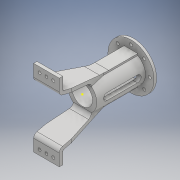
# Autodesk Inventor part: Standard
Saved by Autodesk Inventor 2017 (Build 210142000, 142)
## iProperties
Created: 2018-11-18
Part Number: Standard
Material: Generic
Document SubType Name: Modeling
Designer: Arman Grewal
Density: 1 g/cm^3
Appearance: Default
Author: Arman Grewal
Autodesk Inventor part; units mm, degrees
ref_plane "YZ Plane" through (0, 0, 0) normal (1, 0, 0) x (0, 1, 0)
ref_plane "XZ Plane" through (0, 0, 0) normal (0, 1, 0) x (-1, 0, 0)
sketch "Sketch1" plane through (0, 0, 0) normal (1, 0, 0) x (0, 1, 0)
  line L0 (-60, -12) -> (-60, 12)
  line L1 (-60, -13.0507) -> (-60, -12)
  arc A0 (-37.1036, -17) -> (-48.7347, -18.3716) centre (-37.1036, -67) ccw
  line L2 (-60, -12) -> (-3, -12)
  line L3 (-1, -12) -> (-60, -12)
  line L4 (-3, -17) -> (-37.1036, -17)
  line L5 (-3, 27) -> (-3, -27)
  line L6 (-3, -12) -> (-3, -17)
  line L7 (-102, -45) -> (-102, -30.9493)
  line L8 (-98.1581, -26.0853) -> (-63.8419, -17.9147)
  arc A1 (-63.8419, -17.9147) -> (-60, -13.0507) centre (-65, -13.0507) ccw
  line L9 (-96.4652, -29.788) -> (-48.7347, -18.3716)
  arc A2 (-96.4652, -29.788) -> (-98, -31.7331) centre (-96, -31.7331) ccw
  line L10 (-98, -45) -> (-98, -31.7331)
  arc A3 (-98.1581, -26.0853) -> (-102, -30.9493) centre (-97, -30.9493) ccw
  line L11 (-102, -45) -> (-98, -45)
  point P0 (0, 0)
  point P1 (0, 0)
  point P2 (0, 0)
  point P3 (-43, -17)
  point P4 (-60, -16)
  point P5 (-3, -16)
  point P6 (-102, -27)
  dimension "d0" = 18
  dimension "d1" = 40
  dimension "d2" = 4
  dimension "d3" = 2
  dimension "d4" = 5
  dimension "d5" = 50
  dimension "d6" = 13.451
  dimension "d7" = 166.608
  dimension "d8" = 33
  dimension "d9" = 5
  dimension "d10" = 38
  dimension "d11" = 57
  dimension "d12" = 12
  dimension "d13" = 3
  dimension "d14" = 12
  dimension "d15" = 3
  dimension "d16" = 12
  dimension "d17" = 3
  dimension "d18" = 2
  dimension "d19" = 39
  dimension "d20" = 4
  dimension "d21" = 0
  dimension "d22" = 15
  dimension "d23" = 24
  dimension "d24" = 57
  dimension "d25" = 4
  dimension "d26" = 57
  constraints: 24 end point, 8 point on circle, 8 tangent, 7 point on line, 4 centre point, 2 perpendicular, 2 vertical, 1 equal radius, 1 horizontal, 1 parallel
  measures "d0" distance of L7.start point (-102, -27)
  measures "d1" distance of L4.start point (-43, -17)
  measures "d2" distance of L7.start L10.start
  measures "d3" radius of A2
  measures "d4" radius of A3
  measures "d5" radius of A0
  measures "d6" angle of L3 L9
  measures "d7" angle of L3 L8
  measures "d8" distance between parallel lines of L3 L11
  measures "d9" distance between parallel lines of L3 L4
  measures "d10" distance between parallel lines of L0 L10
  measures "d11" distance between parallel lines of L6 L1
  measures "d12" distance from line of point (0, 0) L3
  measures "d13" distance from line of point (0, 0) L6
  measures "d14" distance from line of point (0, 0) L3
  measures "d15" distance from line of point (0, 0) L6
  measures "d16" distance from line of point (0, 0) L3
  measures "d17" distance from line of point (0, 0) L6
  measures "d18" distance from line of L3.start L6
  measures "d19" distance from line of L5.start L3
  measures "d20" distance from line of point (-3, -16) L3
  measures "d21" distance from line of point (-3, -16) L6
  measures "d22" distance from line of L5.end L3
  measures "d23" distance from line of L0.end L3
  measures "d24" distance from line of L3.end L6
  measures "d25" distance from line of point (-60, -16) L3
  measures "d26" distance from line of point (-60, -16) L6
extrude "Extrusion1" add sketch "Sketch1" along normal mid plane 30
mirror "Mirror1" about plane through (0, 0, 0) normal (0, 0, 1) of "Extrusion1"
sketch "Sketch2" plane through (-15, -3, -12) normal (0, 1, 0) x (1, 0, 0)
  circle A0 centre (15, -12) radius 27
  circle A1 centre (15, -12) radius 12
  dimension "d29" = 54
  dimension "d30" = 24
  dimension "d31" = 0
  constraints: 2 centre point, 2 coincident
  measures "d29" diameter of A0
  measures "d30" diameter of A1
  measures "d31" distance of point (15, -12) A0.centre
extrude "Extrusion2" add sketch "Sketch2" along normal blind 3
sketch "Sketch3" plane through (0, 0, 0) normal (0, 1, 0) x (1, 0, 0)
  circle A0 centre (-22, 0) radius 1.75
  circle A1 centre (-15.5563, -15.5563) radius 1.75
  circle A2 centre (0, -22) radius 1.75
  circle A3 centre (15.5563, -15.5563) radius 1.75
  circle A4 centre (22, 0) radius 1.75
  circle A5 centre (15.5563, 15.5563) radius 1.75
  circle A6 centre (0, 22) radius 1.75
  circle A7 centre (-15.5563, 15.5563) radius 1.75
  arc A8 (-21.9304, -1.7486) -> (-16.7436, -14.2707) centre (0, 0) ccw
  arc A9 (-16.7436, 14.2707) -> (-21.9304, 1.7486) centre (0, 0) ccw
  arc A10 (-1.7486, 21.9304) -> (-14.2707, 16.7436) centre (0, 0) ccw
  arc A11 (14.2707, 16.7436) -> (1.7486, 21.9304) centre (0, 0) ccw
  arc A12 (21.9304, 1.7486) -> (16.7436, 14.2707) centre (0, 0) ccw
  arc A13 (1.7486, -21.9304) -> (14.2707, -16.7436) centre (0, 0) ccw
  dimension "d36" = 3.5
  dimension "d37" = 360
  dimension "d39" = 22
  dimension "d40" = 22
  dimension "d41" = 22
  dimension "d42" = 22
  dimension "d43" = 22
  dimension "d44" = 22
  dimension "d45" = 22
  dimension "d46" = 22
  dimension "d48" = 6.4436
  dimension "d49" = 22
  constraints: 20 point on circle, 10 centre point, 1 coincident, 29 other
  measures "d36" diameter of A0
  measures "d39" radius of A13
  measures "d40" radius of A12
  measures "d41" radius of A11
  measures "d42" radius of A10
  measures "d43" radius of A9
  measures "d44" radius of A8
  measures "d45" distance of point (0, 0) point (22, 0)
  measures "d46" distance of point (0, 0) A12.start
  measures "d48" vertical distance of A5.centre A6.centre
  measures "d49" distance of point (0, 0) A5.centre
extrude "Extrusion3" cut sketch "Sketch3" against normal blind 3
sketch "Sketch4" plane through (0, 0, 0) normal (0, 1, 0) x (1, 0, 0)
  circle A0 centre (0, 0) radius 14
  circle A1 centre (0, 0) radius 12
  dimension "d52" = 28
  dimension "d53" = 24
  dimension "d54" = 0
  constraints: 2 centre point, 2 coincident
  measures "d52" diameter of A0
  measures "d53" diameter of A1
  measures "d54" distance of point (0, 0) A0.centre
extrude "Extrusion4" cut sketch "Sketch4" against normal blind 1
ref_plane "Work Plane1" through (0, 0, -45.25) normal (0, 0, 1) x (1, 0, 0)
sketch "Sketch6" plane through (0, 0, -45.25) normal (0, 0, 1) x (1, 0, 0)
  line L0 (-15, -102) -> (15, -102)
  line L1 (15, -102) -> (15, -88)
  line L2 (15, -96.4652) -> (15, -48.7347)
  line L3 (-15, -98.1581) -> (-15, -102)
  line L4 (-15, -102) -> (-15, -88)
  line L5 (-15, -48.7347) -> (-15, -96.4652)
  line L6 (15, -102) -> (-15, -102)
  line L7 (15, -88) -> (15, -43)
  line L8 (15, -43) -> (-15, -43)
  line L9 (-15, -43) -> (-15, -88)
  line L10 (0, -43) -> (-8, -43)
  line L11 (-8, -43) -> (8, -43)
  line L12 (15, -88) -> (8, -43)
  line L13 (-8, -43) -> (-15, -88)
  line L14 (8, -43) -> (8, -3)
  line L15 (-27, -3) -> (27, -3)
  line L16 (-8, -3) -> (-8, -43)
  line L17 (15, -43) -> (15, -3)
  line L18 (8, -3) -> (-15, -3)
  line L19 (-15, -43) -> (-15, -3)
  line L20 (-8, -43) -> (-8, -3)
  line L21 (-15, -3) -> (-15, -43)
  line L22 (-16.5227, -48) -> (-16.5227, -12)
  line L23 (-8, -43) -> (-15, -43)
  line L24 (-15, -37.1036) -> (-15, -48.7347)
  point P0 (0, 0)
  point P1 (0, 0)
  dimension "d71" = 14
  dimension "d72" = 45
  dimension "d73" = 8
  dimension "d74" = 16
  dimension "d75" = 8.842
  dimension "d76" = 8.842
  dimension "d77" = 8.842
  dimension "d78" = 90
  dimension "d79" = 8.842
  dimension "d80" = 8.842
  dimension "d81" = 8.842
  dimension "d82" = 31.5227
  dimension "d83" = 40
  dimension "d84" = 15
  dimension "d85" = 1.2955
  dimension "d86" = 12
  dimension "d87" = 6.0354
  dimension "d88" = 1.3012
  dimension "d89" = 15
  dimension "d90" = 1.2955
  dimension "d91" = 21.8204
  dimension "d92" = 23.6081
  dimension "d93" = 30.9447
  dimension "d94" = 31.2049
  dimension "d95" = 19.4664
  dimension "d96" = 24.9998
  dimension "d97" = 42
  constraints: 50 end point, 9 point on line, 5 parallel, 3 perpendicular, 2 collinear, 1 horizontal, 1 midpoint, 1 vertical
  measures "d71" distance of L0.end L1.end
  measures "d72" distance of L1.end L17.start
  measures "d73" distance of L10.start L16.end
  measures "d74" distance of L16.end L14.start
  measures "d75" angle of L17 L12
  measures "d76" angle of L17 L13
  measures "d77" angle of L7 L12
  measures "d78" angle of L18 L1
  measures "d79" angle of L5 L12
  measures "d80" angle of L4 L12
  measures "d81" angle of L3 L12
  measures "d82" distance between parallel lines of L17 L22
  measures "d83" distance between parallel lines of L15 L8
  measures "d84" distance from line of point (0, 0) L17
  measures "d85" distance from line of point (0, 0) L12
  measures "d86" distance from line of L15.end L17
  measures "d87" distance from line of L2.end L12
  measures "d88" distance from line of L2.start L12
  measures "d89" distance from line of point (0, 0) L17
  measures "d90" distance from line of point (0, 0) L12
  measures "d91" distance from line of L24.start L12
  measures "d92" distance from line of L24.end L12
  measures "d93" distance from line of L5.end L12
  measures "d94" distance from line of L3.start L12
  measures "d95" distance from line of L22.end L12
  measures "d96" distance from line of L22.start L12
  measures "d97" distance from line of L15.start L17
extrude "Extrusion6" cut sketch "Sketch6" along normal blind 999 contours L12 L8 L7 L2 | L5 L9 L8 L13 | L14 L15 L17 L8 | L8 L19 L15 L16
sketch "Sketch7" plane through (0, -3, 0) normal (0, -1, 0) x (1, 0, 0)
  circle A0 centre (0, 0) radius 12
  circle A1 centre (0, 0) radius 17
  dimension "d100" = 24
  dimension "d101" = 34
  dimension "d102" = 0
  constraints: 2 centre point, 2 coincident
  measures "d100" diameter of A0
  measures "d101" diameter of A1
  measures "d102" distance of point (0, 0) A0.centre
extrude "Extrusion7" add sketch "Sketch7" along normal blind 57
sketch "Sketch5" plane through (0, 0, 0) normal (1, 0, 0) x (0, 1, 0)
  line L0 (-63, -12) -> (-63, 12)
  line L1 (-63, 0) -> (-48, 0)
  line L2 (-48, 0) -> (-12, 0)
  circle A0 centre (-12, 0) radius 4
  circle A1 centre (-48, 0) radius 4
  line L3 (-12, 4) -> (-48, 4)
  line L4 (-48, -4) -> (-12, -4)
  point P0 (0, 0)
  point P1 (0, 0)
  dimension "d57" = 15
  dimension "d58" = 36
  dimension "d59" = 8
  dimension "d60" = 8
  dimension "d61" = 8
  dimension "d62" = 4
  dimension "d63" = 0
  dimension "d64" = 4
  dimension "d65" = 63
  dimension "d66" = 8
  dimension "d67" = 12
  constraints: 10 end point, 4 point on circle, 3 tangent, 2 centre point, 2 coincident, 1 horizontal, 1 midpoint, 1 point on line, 1 vertical
  measures "d57" distance of L1.start L1.end
  measures "d58" distance of L1.end L2.end
  measures "d59" diameter of A0
  measures "d60" diameter of A1
  measures "d61" distance between parallel lines of L4 L3
  measures "d62" distance from line of point (0, 0) L3
  measures "d63" distance from line of point (0, 0) L2
  measures "d64" distance from line of point (0, 0) L3
  measures "d65" distance from line of point (0, 0) L0
  measures "d66" distance from line of L0.end L3
  measures "d67" distance of point (0, 0) L2.end
extrude "Extrusion8" cut sketch "Sketch5" along normal mid plane 60
sketch "Sketch8" plane through (0, 0, 0) normal (1, 0, 0) x (0, 1, 0)
  point P0 (0, 0)
sketch "Sketch9" plane through (-15, -98, 31.7331) normal (0, 1, 0) x (1, 0, 0)
  line L0 (0, -13.2669) -> (30, -13.2669) construction
  line L1 (15, -13.2669) -> (15, -7.2669) construction
  circle A0 centre (15, -7.2669) radius 1.75 construction
  circle A1 centre (15, -7.2669) radius 1.75
  circle A2 centre (23, -7.2669) radius 1.75
  circle A3 centre (7, -7.2669) radius 1.75
  circle A4 centre (15, 70.7331) radius 1.75
  circle A5 centre (7, 70.7331) radius 1.75
  circle A6 centre (23, 70.7331) radius 1.75
  line L2 (0, 76.7331) -> (30, 76.7331) projected
  line L3 (15, 76.7331) -> (15, 63.4663) construction
  line L4 (0, 63.4663) -> (30, 63.4663) construction
  line L5 (30, 76.7331) -> (30, 63.4663) construction
  point P0 (15, 31.7331)
  dimension "d107" = 6
  dimension "d108" = 3.5
  dimension "d109" = 3.5
  dimension "d110" = 8
  dimension "d111" = 6
  dimension "d112" = 3.5
  dimension "d113" = 6
  dimension "d114" = 8
  dimension "d115" = 3.5
  dimension "d116" = 3.5
  dimension "d117" = 3.5
  dimension "d118" = 6
  dimension "d119" = 6
  dimension "d120" = 6
  dimension "d121" = 8
  dimension "d122" = 8
  dimension "d123" = 15
  constraints: 7 centre point, 4 end point, 3 midpoint, 2 coincident, 1 concentric, 1 vertical
  measures "d107" distance of L1.start L1.end
  measures "d108" diameter of A0
  measures "d109" diameter of A2
  measures "d110" distance of A2.centre L1.end
  measures "d111" distance from line of L0 A2.centre
  measures "d112" diameter of A3
  measures "d113" distance from line of L0 A3.centre
  measures "d114" distance of L1.end A3.centre
  measures "d115" diameter of A4
  measures "d116" diameter of A5
  measures "d117" diameter of A6
  measures "d118" distance from line of L2 A5.centre
  measures "d119" distance from line of L2 A4.centre
  measures "d120" distance from line of L2 A6.centre
  measures "d121" distance of A4.centre A6.centre
  measures "d122" distance of A5.centre A4.centre
  measures "d123" distance from line of L5 A4.centre
extrude "Extrusion9" cut sketch "Sketch9" against normal blind 10
sketch "Sketch10" plane through (-10.6444, -60, -13.0507) normal (0, -1, 0) x (1, 0, 0)
  point P0 (10.6444, 13.0507)
body "Solid1"
